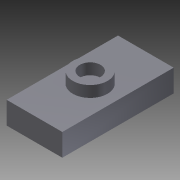
# Autodesk Inventor part: 3794
Saved by Autodesk Inventor 2011 SP1 (Build 150282100, 282)
## iProperties
Company: Allseas Engineering BV
Created: 2011-09-26
Part Number: 3794
Cost Center: 0 kg
Material: Steel
Document SubType Name: Modeling
Designer: PMe
Authority: 0 mm^3
Stock Number: =<Filenr>_<Document number>
Density: 7.85 g/cm^3
Act. Code: DW000
SaveDate: 2011-07-28
SaveTime: 18:32
FileName: Standard
TotalMass: 0 kg
TotalVolume: 0 mm^3
Subject: =<Title><TITLE 1_2> <TITLE 2_2>
Author: PMe
Autodesk Inventor part; units mm, degrees
ref_plane "YZ Plane" through (0, 0, 0) normal (1, 0, 0) x (0, 1, 0)
ref_plane "XZ Plane" through (0, 0, 0) normal (0, 1, 0) x (-1, 0, 0)
ref_plane "XY Plane" through (0, 0, 0) normal (0, 0, 1) x (1, 0, 0)
sketch "Sketch1" plane through (0, 0, 0) normal (0, 0, 1) x (1, 0, 0)
  line L0 (-4, 8) -> (4, 8)
  line L1 (4, 8) -> (4, -8)
  line L2 (4, -8) -> (-4, -8)
  line L3 (-4, -8) -> (-4, 8)
  point P0 (0, 0)
  dimension "d0" = 8
  dimension "d1" = 16
  dimension "d2" = 4
  dimension "d3" = 8
  constraints: 8 end point, 2 parallel, 1 horizontal, 1 perpendicular
  measures "d0" distance of L1.end L2.end
  measures "d1" distance of L0.end L1.end
  measures "d2" distance from line of point (0, 0) L1
  measures "d3" distance from line of point (0, 0) L2
extrude "Extrusion1" add sketch "Sketch1" along normal blind 3.2
shell "Shell1" thickness 1.5 removed faces 1 at (-1.3333, 2.6667, 0)
sketch "Sketch2" plane through (0, 0, 3.2) normal (0, 0, 1) x (1, 0, 0)
  circle A0 centre (0, -4) radius 2.5
  line L0 (4, 8) -> (4, -8) projected
  line L1 (4, -8) -> (-4, -8) projected
  dimension "d7" = 5
  dimension "d10" = 4
  dimension "d11" = 4
  constraints: 1 centre point, 1 coincident
  measures "d7" diameter of A0
  measures "d10" distance from line of L1 point (0, -4)
  measures "d11" distance from line of L0 point (0, -4)
extrude "Extrusion2" [suppressed]
sketch "Sketch3" plane through (2.5, -6.5, 1.7) normal (0, 0, -1) x (-1, 0, 0)
  point P0 (2.5, 6.5)
extrude "Extrusion3" [suppressed]
pattern_linear "Rectangular Pattern1" [suppressed]
sketch "Sketch4" plane through (2.5, -6.5, 1.7) normal (0, 0, -1) x (-1, 0, 0)
  point P0 (2.5, 6.5)
extrude "Extrusion4" [suppressed]
pattern_linear "Rectangular Pattern2" [suppressed]
sketch "Sketch5" plane through (0, 0, 3.2) normal (0, 0, 1) x (1, 0, 0)
  circle A0 centre (0, 0) radius 2.5
  circle A1 centre (0, 0) radius 1.5
  dimension "d41" = 5
  dimension "d42" = 3
  constraints: 2 centre point, 2 coincident
  measures "d41" diameter of A0
  measures "d42" diameter of A1
extrude "Extrusion5" add sketch "Sketch5" along normal blind 1.6
equation "\"d0\" = 8 * WIDTH"
equation "\"d1\" = 8 * LENGTH"
equation "\"d2\" = 0.5 * d0"
equation "\"d3\" = 0.5 * d1"
equation "\"d4\" = HEIGHT"
equation "\"WIDTH\" = 1"
equation "\"HEIGHT\" = 3.2"
equation "\"LENGTH\" = 2"
body "Solid1"
